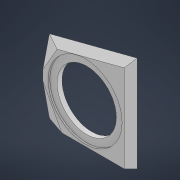
# Autodesk Inventor part: Front1
Saved by Autodesk Inventor 2022 (Build 260153000, 153)
## iProperties
Created: 2022-04-08
Part Number: Front1
Material: Типовые
Document SubType Name: Modeling
Designer: Kalugin_a
Density: 1 g/cm^3
Appearance: По умолчанию
Author: Kalugin_a
Autodesk Inventor part; units mm, degrees
ref_plane "YZ Plane" through (0, 0, 0) normal (1, 0, 0) x (0, 1, 0)
sketch "Эскиз1" plane through (0, 0, 0) normal (0, 0, 1) x (1, 0, 0)
  line L0 (0, 0) -> (216, 0)
  circle A0 centre (104, 96) radius 73
  circle A1 centre (104, 96) radius 91
  line L1 (0, 180) -> (216, 236)
  line L2 (0, 87) -> (48, 0) construction
  line L3 (0, 0) -> (0, 180)
  line L4 (216, 236) -> (216, 0)
  line L5 (48, 192.4444) -> (0, 112) construction
  point P0 (43.1585, 192.0844)
  point P1 (92.1531, 205.8029)
  dimension "d2" = 146
  dimension "d3" = 182
  dimension "d6" = 236
  dimension "d7" = 180
  dimension "d8" = 96
  dimension "d15" = 48
  dimension "d16" = 48
  dimension "d17" = 87
  dimension "d18" = 68
  dimension "d22" = 216
  constraints: 12 end point, 3 coincident, 3 point on line, 2 centre point, 1 horizontal, 1 parallel, 1 vertical
  measures "d2" diameter of A0
  measures "d3" diameter of A1
  measures "d6" distance of L0.end L1.end
  measures "d7" distance of L0.start L1.start
  measures "d8" distance from line of L0 A0.centre
  measures "d15" distance of point (48, 0) point (0, 0)
  measures "d16" horizontal distance of L5.start L1.start
  measures "d17" distance of point (0, 0) point (0, 87)
  measures "d18" distance of L5.end L1.start
  measures "d22" distance of L0.end point (0, 0)
extrude "Выдавливание2" add sketch "Эскиз1" along normal blind 12 contours A1
extrude "Выдавливание3" add sketch "Эскиз1" along normal blind 16 contours L3 L1 L4 L0
sketch "Эскиз4" plane through (0, 0, 0) normal (-1, 0, 0) x (0, 0, 1)
  line L0 (16, 180) -> (16, 0) projected
  point P0 (0, 0)
  point P1 (16, 87)
  point P2 (16, 112)
  dimension "d19" = 87
  dimension "d20" = 68
  constraints: 2 point on line
  measures "d19" distance of L0.end point (16, 87)
  measures "d20" distance of point (16, 112) L0.start
sketch "Эскиз5" plane through (0, 180, 16) normal (-0.2509622, 0.9679969, 0) x (0.9679969, 0.2509622, 0)
  line L0 (223.1412, 0) -> (0, 0) projected
  point P0 (-45.1732, 16)
  point P1 (48, 0)
  dimension "d21" = 48
  constraints: 1 point on line
  measures "d21" distance of L0.end point (48, 0)
ref_plane "РабПлоскость1" through (46.4639, 192.0462, 16) normal (-0.3670406, 0.2130535, 0.9054774) x (-0.9183225, -0.2380836, -0.3162278)
split "Разделение1" plane through (46.4639, 192.0462, 16) removes the side toward (-0.3670406, 0.2130535, 0.9054774)
sketch "Эскиз6" plane through (0, 0, 0) normal (0, -1, 0) x (1, 0, 0)
  line L0 (216, 16) -> (46.4639, 16) projected
  point P0 (0, 0)
ref_plane "РабПлоскость2" through (46.4639, 0, 16) normal (0.3207767, 0.1713163, -0.9315326) x (-0.945511, 0, -0.3255902)
split "Разделение2" plane through (46.4639, 0, 16) removes the side toward (-0.3207767, -0.1713163, 0.9315326)
chamfer "Фаска1" distance 16 angle 45 2 edges at (216, 118, 16) (131.2319, 214.0231, 16)
